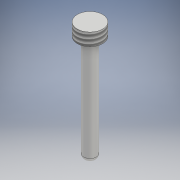
# Autodesk Inventor part: Structure_SwitchPin
Saved by Autodesk Inventor 2018 (Build 220112000, 112)
## iProperties
Created: 2019-03-30
Part Number: Structure_SwitchPin
Material: Stainless Steel
Document SubType Name: Modeling
Designer: Bradley
Density: 8 g/cm^3
Appearance: Semi-Polished
Author: Bradley
Autodesk Inventor part; units mm, degrees
ref_plane "YZ Plane" through (0, 0, 0) normal (1, 0, 0) x (0, 1, 0)
ref_plane "XZ Plane" through (0, 0, 0) normal (0, 1, 0) x (-1, 0, 0)
ref_plane "XY Plane" through (0, 0, 0) normal (0, 0, 1) x (1, 0, 0)
sketch "Sketch1" plane through (0, 0, 0) normal (0, 1, 0) x (-1, 0, 0)
  line L0 (0, 7) -> (-1.5, 7)
  line L1 (-1.5, 7) -> (-1.5, 5.5)
  line L2 (-1.5, 5.5) -> (-0.75, 5.5)
  line L3 (-0.75, 5.5) -> (-0.75, -6.5)
  line L4 (0, -7) -> (0, 7)
  arc A0 (-0.75, -6.5) -> (-0.25, -7) centre (-0.25, -6.5) ccw
  line L5 (-0.25, -7) -> (0, -7)
  point P0 (0, 0)
  point P1 (0, 0)
  dimension "d0" = 3
  dimension "d1" = 1.5
  dimension "d2" = 12.5
  dimension "d3" = 0.5
  dimension "d4" = 1.5
  constraints: 12 end point, 4 perpendicular, 2 point on circle, 2 tangent, 1 centre point, 1 coincident, 1 horizontal, 1 midpoint, 1 parallel
  measures "d0" diameter of L1 L4
  measures "d1" diameter of L3 L4
  measures "d2" distance between parallel lines of L2 L5
  measures "d3" radius of A0
  measures "d4" distance of L0.end L1.end
revolve "Revolution1" add sketch "Sketch1" angle 360 about axis through (0, 0, -7) along (0, 0, 1)
thread "Thread1" size "M3x0.5" class "6g" standard "ANSI Metric M Profile" full length
body "Solid1"
